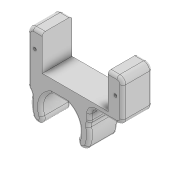
# Autodesk Inventor part: frame_2
Saved by Autodesk Inventor 2022 (Build 260153000, 153)
## iProperties
Created: 2023-05-17
Part Number: frame_2
Material: 일반
Document SubType Name: Modeling
Designer: HCI-TECH_KDK
Density: 1 g/cm^3
Appearance: 기본값
Author: HCI-TECH_KDK
Autodesk Inventor part; units mm, degrees
ref_plane "YZ Plane" through (0, 0, 0) normal (1, 0, 0) x (0, 1, 0)
ref_plane "XZ Plane" through (0, 0, 0) normal (0, 1, 0) x (-1, 0, 0)
ref_plane "XY Plane" through (0, 0, 0) normal (0, 0, 1) x (1, 0, 0)
sketch "스케치1" plane through (0, 0, 0) normal (0, 0, 1) x (1, 0, 0)
  line L0 (0, 0) -> (22.2, 0)
  line L1 (22.2, 0) -> (22.2, 11.8)
  line L2 (22.2, 11.8) -> (0, 11.8)
  line L3 (0, 11.8) -> (0, 0)
  circle A0 centre (6, 5.9) radius 1.8779
  line L4 (-9, 5.9) -> (21, 5.9)
  line L5 (21, 5.9) -> (21, -16.1)
  line L6 (21, -16.1) -> (-9, -16.1)
  line L7 (-9, -16.1) -> (-9, 5.9)
  line L8 (-24.5431, -4.6) -> (59.0522, -4.6) construction
  line L9 (-2, 5.9) -> (14, 5.9) construction
  line L10 (14, 5.9) -> (14, -16.1) construction
  line L11 (14, -16.1) -> (-2, -16.1) construction
  line L12 (-2, -16.1) -> (-2, 5.9) construction
  line L13 (-5, 11.8) -> (27.2, 11.8)
  line L14 (27.2, 11.8) -> (27.2, 0)
  line L15 (27.2, 0) -> (-5, 0)
  line L16 (-5, 0) -> (-5, 11.8)
  point P0 (6, 5.9)
  point P1 (6, 5.9)
  point P2 (0, 5.9)
  point P3 (11.1, 11.8)
  point P4 (11.1, 11.8)
  dimension "d0" = 22.2
  dimension "d1" = 11.8
  dimension "d2" = 6
  dimension "d3" = 22
  dimension "d4" = 30
  dimension "d5" = 11.5
  dimension "d6" = 16
  dimension "d10" = 32.2
  constraints: 34 end point, 8 parallel, 5 horizontal, 5 midpoint, 4 coincident, 4 perpendicular, 2 point on line, 1 centre point, 1 horizontal alignment
  measures "d0" distance of L1.end L2.end
  measures "d1" distance of L0.end L1.end
  measures "d2" distance from line of L3 A0.centre
  measures "d3" distance of L4.end L5.end
  measures "d4" distance of L5.end L6.end
  measures "d5" distance between parallel lines of L6 L8
  measures "d6" distance between parallel lines of L12 L10
  measures "d10" distance of L13.start L13.end
sketch "스케치2" plane through (0, 0, 0) normal (0, 0, 1) x (1, 0, 0)
  line L0 (-24.5431, -4.6) -> (59.0522, -4.6) construction
  line L1 (-2, -16.1) -> (-2, 5.9) construction
  line L2 (14, 5.9) -> (14, -16.1) construction
  line L3 (21, -16.1) -> (-9, -16.1) projected
  line L4 (-2, -4.6) -> (14, -4.6)
  line L5 (14, -4.6) -> (14, -16.1)
  line L6 (14, -16.1) -> (-2, -16.1)
  line L7 (-2, -16.1) -> (-2, -4.6)
  line L8 (-4, -18.1) -> (16, -18.1)
  line L9 (16, -18.1) -> (16, -2.6)
  line L10 (16, -2.6) -> (-4, -2.6)
  line L11 (-4, -2.6) -> (-4, -18.1)
  point P0 (0, 0)
  point P1 (-2, -16.1)
  dimension "d7" = 2
  dimension "d42" = 11.5
  dimension "d43" = 16
  constraints: 16 end point, 4 parallel, 2 perpendicular, 2 point on line, 1 horizontal, 3 other
  measures "d7" distance between parallel lines of L6 L8
  measures "d42" distance of L6.end L4.start
  measures "d43" distance between parallel lines of L2 L1
extrude "돌출1" add sketch "스케치2" against normal blind 10 contours L3 L9 L8 L11 | L5 L4 L7 L3 L11 L10 L9
sketch "스케치3" plane through (0, 0, 0) normal (0, 0, 1) x (1, 0, 0)
  line L0 (0, 11.8) -> (0, 0) projected
  line L1 (-5, 11.8) -> (27.2, 11.8) projected
  line L2 (-5, 0) -> (-5, 11.8) projected
  line L3 (27.2, 0) -> (-5, 0) projected
  line L4 (27.2, 11.8) -> (27.2, 0) projected
  line L5 (22.2, 0) -> (22.2, 11.8) projected
  line L6 (27.2, 11.8) -> (22.2, 11.8)
  line L7 (27.2, 0) -> (27.2, -6.5936)
  line L8 (27.2, -6.5936) -> (16, -6.5936)
  line L9 (16, -2.6) -> (16, -18.1) projected
  line L10 (-9, -16.1) -> (-9, 5.9) projected
  line L11 (-4, -18.1) -> (-4, -2.6) projected
  line L12 (-4, -6.5936) -> (-9, -6.5936)
  line L13 (-9, 5.9) -> (0, 5.9)
  line L14 (21, 5.9) -> (21, -16.1) projected
  line L15 (0, 0) -> (22.2, 0) projected
  line L16 (16, -2.6) -> (-4, -2.6) projected
  line L17 (16, -18.1) -> (16, -2.6) projected
  point P0 (-5, 5.9)
  constraints: 10 end point, 3 point on line, 2 perpendicular, 1 collinear, 1 midpoint, 1 vertical
extrude "돌출2" add sketch "스케치3" against normal blind 10 contours L0 L13 L2 L1 | L0 L3 L2 L13 | L1 L4 L3 L5 | L3 L14 L8 L9 L16 L11 L12 L10 L13 L2 | L3 L7 L8 L14
sketch "스케치4" plane through (0, 0, 0) normal (0, 0, 1) x (1, 0, 0)
  line L0 (-5, 11.8) -> (27.2, 11.8) projected
  line L1 (-5, 11.8) -> (-5, 5.9) projected
  line L2 (-5, 0) -> (-5, 11.8) projected
  line L3 (27.2, 0) -> (-5, 0) projected
  line L4 (27.2, -6.5936) -> (27.2, 11.8) projected
  line L5 (27.2, 11.8) -> (22.2, 11.8) projected
  line L6 (22.2, 11.8) -> (0, 11.8) projected
  line L7 (-5, 11.8) -> (0, 11.8)
  line L8 (0, 11.8) -> (0, 0)
  line L9 (0, 0) -> (-5, 0)
  line L10 (-5, 0) -> (-5, 11.8)
  line L11 (22.2, 11.8) -> (27.2, 11.8)
  line L12 (27.2, 11.8) -> (27.2, 0)
  line L13 (27.2, 0) -> (22.2, 0)
  line L14 (22.2, 0) -> (22.2, 11.8)
  circle A0 centre (-2.5, 5.9) radius 0.5
  circle A1 centre (24.7, 5.9) radius 0.5
  dimension "d13" = 1
  dimension "d14" = 1
  constraints: 16 end point, 4 parallel, 2 centre point, 2 horizontal, 2 perpendicular
  measures "d13" diameter of A0
  measures "d14" diameter of A1
extrude "돌출3" cut sketch "스케치4" against normal blind 6 contours A0 | A1
sketch "스케치16" plane through (-9, 5.9, 0) normal (0, 1, 0) x (1, 0, 0)
  line L0 (4, 0) -> (0, 0) projected
  line L1 (4, 0) -> (4, 10) projected
  line L2 (0, 10) -> (4, 10) projected
  line L3 (0, 0) -> (0, 10) projected
  point P0 (9, 0)
extrude "돌출11" cut sketch "스케치16" against normal blind 32.25
sketch "스케치17" plane through (27.2, -6.5936, 0) normal (1, 0, 0) x (0, 0, -1)
  line L0 (0, 1.9936) -> (10, 1.9936) projected
  line L1 (0, 0) -> (10, 0) projected
  line L2 (10, 18.3936) -> (10, 0) projected
  line L3 (0, 0) -> (10, 0)
  line L4 (10, 0) -> (10, 4.42)
  line L5 (10, 4.42) -> (0, 4.42)
  line L6 (0, 4.42) -> (0, 0)
  point P0 (0, 6.5936)
  constraints: 8 end point, 2 parallel, 1 horizontal, 1 perpendicular, 1 point on line
extrude "돌출12" cut sketch "스케치17" against normal blind 11.2
sketch "Sketch18" plane through (0, 0, 0) normal (0, 0, 1) x (1, 0, 0)
  point P0 (0, 0)
sketch "Sketch20" plane through (0, 0, 0) normal (0, 0, 1) x (1, 0, 0)
  line L0 (16, -2.1737) -> (27.2, -2.1737) projected
  line L1 (27.2, -2.1737) -> (27.2, 11.8) projected
  line L2 (27.2, 11.8) -> (22.2, 11.8) projected
  line L3 (22.2, 11.8) -> (22.2, 0) projected
  line L4 (22.2, 0) -> (0, 0) projected
  line L5 (0, 0) -> (0, 11.8) projected
  line L6 (0, 11.8) -> (-5, 11.8) projected
  line L7 (-5, 11.8) -> (-5, -6.5936) projected
  line L8 (-5, -6.5936) -> (-4, -6.5936) projected
  line L9 (-4, -6.5936) -> (-4, -18.1) projected
  line L10 (-4, -18.1) -> (16, -18.1) projected
  line L11 (16, -18.1) -> (16, -2.1737) projected
  line L12 (-2, -16.1) -> (-2, -4.6) projected
  line L13 (-2, -4.6) -> (14, -4.6) projected
  line L14 (14, -4.6) -> (14, -16.1) projected
  line L15 (14, -16.1) -> (-2, -16.1) projected
  circle A0 centre (24.7, 5.9) radius 0.5 projected
  circle A1 centre (-2.5, 5.9) radius 0.5 projected
  line L16 (-4, -6.5936) -> (-5, -6.5936) projected
  line L17 (-5, -6.5936) -> (16, -6.5936)
  line L18 (16, -2.1737) -> (16, -18.1) projected
  point P0 (14, -6.5936)
  point P1 (-2, -6.5936)
  constraints: 2 end point, 1 perpendicular, 1 point on line
extrude "Extrusion13" cut sketch "Sketch20" against normal blind 10 contours L11 L10 L9 L17 L12 L15 L14
sketch "Sketch21" plane through (0, 0, 0) normal (0, 0, 1) x (1, 0, 0)
  arc A0 (11.2137, -14.2419) -> (0.5647, -14.2419) centre (5.8892, -10.5136) ccw
  arc A1 (14.1116, -16.2711) -> (-2.3333, -16.2711) centre (5.8892, -10.5136) ccw
  line L0 (5.8892, -10.5136) -> (-2.3333, -16.2711)
  line L1 (5.8892, -10.5136) -> (14.1116, -16.2711)
  line L2 (5.8892, -10.5136) -> (5.8892, 0)
  line L3 (0, 0) -> (22.2, 0) projected
  line L4 (-5, -6.5936) -> (-2, -6.5936) projected
  line L5 (-2, -6.5936) -> (-2, -4.6) projected
  line L6 (-2, -4.6) -> (14, -4.6) projected
  line L7 (14, -4.6) -> (14, -6.5936) projected
  line L8 (14, -6.5936) -> (16, -6.5936) projected
  line L9 (16, -6.5936) -> (16, -2.1737) projected
  line L10 (16, -2.1737) -> (27.2, -2.1737) projected
  line L11 (27.2, -2.1737) -> (27.2, 11.8) projected
  line L12 (27.2, 11.8) -> (22.2, 11.8) projected
  line L13 (22.2, 11.8) -> (22.2, 0) projected
  line L14 (22.2, 0) -> (0, 0) projected
  line L15 (0, 0) -> (0, 11.8) projected
  line L16 (0, 11.8) -> (-5, 11.8) projected
  line L17 (-5, 11.8) -> (-5, -6.5936) projected
  circle A2 centre (24.7, 5.9) radius 0.5 projected
  circle A3 centre (-2.5, 5.9) radius 0.5 projected
  dimension "d53" = 13
  dimension "d54" = 125
  dimension "d55" = 125
  constraints: 6 end point, 5 point on circle, 3 point on line, 2 centre point, 1 vertical
  measures "d53" diameter of A0
  measures "d54" angle of L2 L1
  measures "d55" angle of L2 L0
extrude "Extrusion14" add sketch "Sketch21" against normal blind 10 contours A0 L6 L7 L8 A1 L1 | A0 L2 A1 L6 | A0 L6 L5 L4 A1 L2 | A1 L8 L7 | L0 A1 L4 L5 L6 A0
fillet "Fillet6" radius 2 12 edges at (0.5647, -14.2419, -5) (-2.3333, -16.2711, -5) (11.2137, -14.2419, -5) (14.1116, -16.2711, -5) (-5, -6.5936, -5) (-3.3515, -6.5936, -5) (16, -6.5936, -5) (15.1299, -6.5936, -5) (27.2, -2.1737, -5) (16, -2.1737, -5) (27.2, 11.8, -5) (-5, 11.8, -5)
fillet "Fillet7" radius 1 46 edges at (16.5858, -2.7594, -10) (16, -5.1162, -10) (15.9509, -6.4993, -10) (15.6234, -7.5632, -10) (15.9034, -11.201, -10) (14.1972, -15.2244, -10) (26.6142, -1.5879, -10) (27.2, 4.8132, -10) (26.6142, 11.2142, -10) (23.7, 11.8, -10) (21.6, -2.1737, -10) (-4.8645, -6.3774, -10) (-5, 2.0731, -10) (-4.4142, 11.2142, -10) (-1.5, 11.8, -10) (-4.1053, -11.4449, -10) (-2.4188, -15.2244, -10) (-4.0307, -7.7995, -10) (26.6142, 11.2142, 0) (23.7, 11.8, 0) (26.6142, -1.5879, 0) (21.6, -2.1737, 0) (16.5858, -2.7594, 0) (16, -5.1162, 0) (15.9509, -6.4993, 0) (15.6234, -7.5632, 0) (15.9034, -11.201, 0) (14.1972, -15.2244, 0) (27.2, 4.8132, 0) (-4.8645, -6.3774, 0) (-4.0307, -7.7995, 0) (-4.1053, -11.4449, 0) (-2.4188, -15.2244, 0) (-4.4142, 11.2142, 0) (-1.5, 11.8, 0) (-5, 2.0731, 0) (-0.1107, -14.1921, 0) (-0.1357, -8.0742, 0) (5.8892, -4.6, 0) (11.8891, -14.1921, 0) (11.9141, -8.0742, 0) (5.8892, -4.6, -10) (-0.1107, -14.1921, -10) (-0.1357, -8.0742, -10) (11.8891, -14.1921, -10) (11.9141, -8.0742, -10)
